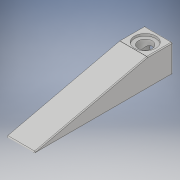
# Autodesk Inventor part: Wedge_base-left
Saved by Autodesk Inventor 2019.3 (Build 233278000, 278)
## iProperties
Created: 2019-02-07
Part Number: Wedge_base-left
Material: Generic
Document SubType Name: Modeling
Designer: Varga Daniel
Density: 1 g/cm^3
Appearance: Default
Author: Varga Daniel
Autodesk Inventor part; units mm, degrees
ref_plane "YZ Plane" through (0, 0, 0) normal (1, 0, 0) x (0, 1, 0)
ref_plane "XZ Plane" through (0, 0, 0) normal (0, 1, 0) x (-1, 0, 0)
ref_plane "XY Plane" through (0, 0, 0) normal (0, 0, 1) x (1, 0, 0)
derived "Connector_pin_base.ipt"
sketch "Pin_base_sketch" plane through (0, 0, 0) normal (0, 0, 1) x (1, 0, 0)
  line L0 (0, 0) -> (23.0918, 0) construction
  line L1 (0, 0) -> (0, 6.22) construction
  line L2 (0, 3.75) -> (0.563, 3.75)
  line L3 (0.863, 3.45) -> (0.863, 2.475)
  line L4 (0.863, 2.475) -> (9.988, 2.475)
  line L5 (9.988, 2.475) -> (9.988, 0)
  line L6 (0, 0) -> (0, 3.75)
  line L7 (0, 0) -> (9.988, 0)
  line L8 (9.288, 2.475) -> (9.288, 2.6)
  line L9 (9.988, 2.475) -> (9.988, 2.4774)
  arc A0 (9.988, 2.4774) -> (9.8454, 2.7031) centre (9.738, 2.4774) ccw
  arc A1 (9.8454, 2.7031) -> (9.288, 2.6) centre (9.6379, 2.267) ccw
  line L10 (9.8454, 2.7031) -> (9.8454, -0.0362) construction
  line L11 (8.9584, 2.75) -> (10.3858, 2.75) construction
  arc A2 (0.863, 3.45) -> (0.563, 3.75) centre (0.563, 3.45) ccw
  line L12 (0.863, 2.475) -> (0.863, 0)
  line L13 (-0.863, 2.475) -> (-0.863, 0)
  line L14 (-0.863, 3.45) -> (-0.863, 2.475)
  arc A3 (-0.563, 3.75) -> (-0.863, 3.45) centre (-0.563, 3.45) ccw
  line L15 (0, 3.75) -> (-0.563, 3.75)
  line L16 (0, 0) -> (-23.0918, 0) construction
  line L17 (0, 0) -> (-9.988, 0)
  line L18 (-0.863, 2.475) -> (-9.988, 2.475)
  line L19 (-9.288, 2.475) -> (-9.288, 2.6)
  arc A4 (-9.288, 2.6) -> (-9.8454, 2.7031) centre (-9.6379, 2.267) ccw
  arc A5 (-9.8454, 2.7031) -> (-9.988, 2.4774) centre (-9.738, 2.4774) ccw
  line L20 (-9.988, 2.475) -> (-9.988, 2.4774)
  line L21 (-8.9584, 2.75) -> (-10.3858, 2.75) construction
  line L22 (-9.8454, 2.7031) -> (-9.8454, -0.0362) construction
  line L23 (-9.988, 2.475) -> (-9.988, 0)
  line L24 (9.638, 3.1946) -> (9.638, -1.2485) construction
  dimension "d18" = 7.5
  dimension "d19" = 0.3
  dimension "d52" = 8.425
  dimension "d53" = 9.988
  measures "d18" diameter of L2 L0
  measures "d19" radius of A2
  measures "d52" distance between parallel lines of L19 L14
  measures "d53" distance between parallel lines of L23 L1
derived "Base_part.ipt"
sketch "Beam_sketch" plane through (0, 0, 0) normal (0, 1, 0) x (-1, 0, 0)
  line L0 (5, 0) -> (25, 0)
  line L1 (30, 5) -> (30, 25)
  line L2 (25, 30) -> (5, 30)
  line L3 (0, 25) -> (0, 5)
  line L4 (5, 29) -> (25, 29)
  line L5 (29, 25) -> (29, 5)
  line L6 (25, 1) -> (5, 1)
  line L7 (1, 5) -> (1, 25)
  circle A0 centre (5, 5) radius 2.5
  circle A1 centre (5, 5) radius 3.5
  arc A2 (25, 0) -> (30, 5) centre (25, 5) ccw
  arc A3 (30, 25) -> (25, 30) centre (25, 25) ccw
  arc A4 (5, 30) -> (0, 25) centre (5, 25) ccw
  arc A5 (0, 5) -> (5, 0) centre (5, 5) ccw
  arc A6 (1, 5) -> (5, 1) centre (5, 5) ccw
  arc A7 (5, 29) -> (1, 25) centre (5, 25) ccw
  arc A8 (29, 25) -> (25, 29) centre (25, 25) ccw
  arc A9 (25, 1) -> (29, 5) centre (25, 5) ccw
  line L8 (49.1041, 15) -> (-27.081, 15) construction
  line L9 (31.1478, 10) -> (-2.4877, 10) construction
  line L10 (-2.8604, 5) -> (35.495, 5) construction
  line L11 (5, -2.5736) -> (5, 36.7522) construction
  line L12 (15, -1.4978) -> (15, 34.8784) construction
  line L13 (1.5359, 5.5) -> (1, 5.5)
  line L14 (1.5359, 4.5) -> (1.0314, 4.5)
  line L15 (28.9686, 4.5) -> (8.4641, 4.5)
  line L16 (29, 5.5) -> (8.4641, 5.5)
  line L17 (4.5, 1.5359) -> (4.5, 1.0314)
  line L18 (5.5, 1.5359) -> (5.5, 1)
  line L19 (29, 10.5) -> (1, 10.5)
  line L20 (29, 9.5) -> (1, 9.5)
  line L21 (4.5, 28.9686) -> (4.5, 10.5)
  line L22 (4.5, 9.5) -> (4.5, 8.4641)
  line L23 (5.5, 29) -> (5.5, 10.5)
  line L24 (5.5, 9.5) -> (5.5, 8.4641)
  point P0 (0, 0)
  point P1 (30, 30)
  point P2 (0, 30)
  dimension "d1" = 7
  dimension "d2" = 5
  measures "d2" diameter of A0
sketch "Sketch2" plane through (0, 0, 0) normal (1, 0, 0) x (0, 1, 0)
  line L0 (0, 0) -> (10, 0)
  line L1 (10, 0) -> (10, 9.2)
  line L2 (10, 9.2) -> (0.5922, 49.7678)
  line L3 (0, 49.7) -> (0, 0)
  line L4 (0, 47.895) -> (8.9735, 9.2)
  line L5 (8.9735, 9.2) -> (0, 9.2)
  arc A0 (0.5922, 49.7678) -> (0, 49.7) centre (0.3, 49.7) ccw
  point P0 (0, 52.3216)
  dimension "d3" = 10
  dimension "d5" = 1
  dimension "d6" = 9.2
  dimension "d38" = 0.3
  dimension "d39" = 50
  constraints: 12 end point, 5 point on line, 2 parallel, 2 perpendicular, 2 point on circle, 2 tangent, 1 centre point, 1 horizontal
  measures "d3" distance between parallel lines of L1 L3
  measures "d5" distance between parallel lines of L2 L4
  measures "d6" distance between parallel lines of L5 L0
  measures "d38" radius of A0
extrude "Extrusion1" add sketch "Sketch2" against normal blind 10 contours L3 L5 L4 A0 L2 L1 L0
extrude "Left_wall" add sketch "Sketch2" against normal blind 1 contours L3 L4 L5
sketch "Sketch3" plane through (-10, 0, 0) normal (-1, 0, 0) x (0, 0, 1)
  line L0 (9.2, 8.9735) -> (9.2, 0) projected
  line L1 (47.895, 0) -> (9.2, 8.9735) projected
  line L2 (49.7, 0) -> (0, 0) projected
  point P0 (50, 0)
extrude "Right_wall" [suppressed]
sketch "Sketch4" plane through (-10, 0, 0) normal (0, -1, 0) x (1, 0, 0)
  line L0 (9, 47.895) -> (0, 47.895) construction
  line L1 (9, 9.2) -> (0, 9.2) construction
  line L2 (10, 0) -> (0, 0) construction
  line L3 (10, 49.7) -> (10, 0) construction
  circle A0 centre (5, 5) radius 3.85
  circle A1 centre (5, 5) radius 2.5
  line L4 (10, 49.7) -> (0, 49.7) projected
  line L5 (0, 47.895) -> (0, 49.7) projected
  line L6 (9, 9.2) -> (9, 47.895) projected
  line L7 (0, 0) -> (0, 9.2) projected
  dimension "d14" = 5
  dimension "d15" = 5
  dimension "d16" = 7.7
  dimension "d49" = 5
  constraints: 2 centre point, 1 coincident
  measures "d14" distance from line of A0.centre L2
  measures "d15" diameter of A1
  measures "d16" diameter of A0
  measures "d49" distance from line of A0.centre L3
extrude "Extrusion4" cut sketch "Sketch4" against normal through all contours A1
extrude "Extrusion6" cut sketch "Sketch4" against normal blind 0.8
sketch "Sketch6" plane through (0, 10, 9.2) normal (0, 1, 0) x (1, 0, 0)
  circle A0 centre (-5, 4.2) radius 3.85 projected
  circle A1 centre (-5, 4.2) radius 2.5 projected
  point P0 (0, 9.2)
extrude "Extrusion7" cut sketch "Sketch6" against normal blind 0.8
sketch "Sketch10" plane through (0, 0, 0) normal (0, 0, -1) x (-1, 0, 0)
  line L0 (0, 0) -> (0, 10) construction
  line L1 (0, 0) -> (10, 0) construction
  line L2 (10, 10) -> (10, 0) construction
  line L3 (0, 10) -> (10, 10) construction
  circle A0 centre (5, 5) radius 2.5
  circle A1 centre (5, 5) radius 3.85
  dimension "d43" = 5
  dimension "d44" = 7.7
  dimension "d45" = 5
  dimension "d46" = 5
  constraints: 2 centre point, 1 coincident
  measures "d43" diameter of A0
  measures "d44" diameter of A1
  measures "d45" distance from line of A0.centre L2
  measures "d46" distance from line of A0.centre L1
extrude "Extrusion11" cut sketch "Sketch10" against normal up to surface (9.2 mm away) contours A0
extrude "Extrusion12" cut sketch "Sketch10" against normal blind 0.8
fillet "Fillet1" radius 0.3 3 edges at (-5, 10, 0) (-5, 0, 0) (-5, 10, 9.2)
fillet "Left_fillet" radius 0.3 8 edges at (0, 9.9981, 9.1998) (0, 5.2922, 29.5006) (0, 0.2659, 49.9981) (0, 0, 25) (0, 0.0879, 0.0879) (0, 5, 0) (0, 9.9121, 0.0879) (0, 10, 4.7328)
fillet "Right_fillet" [suppressed]
equation "\"d5\" = Wall_thickness"
equation "\"d6\" = 0.5 * Overall_height + 0.5 * Hole_height"
equation "\"d38\" = Wedge_end_fillet_radius"
equation "\"d39\" = Wedge_length"
equation "\"d9\" = Wall_thickness"
equation "\"d11\" = Wall_thickness"
equation "\"d15\" = d2"
equation "\"d16\" = d18 + Wedge_Pin_collar_diameter_tolerance"
equation "\"d20\" = Wall_thickness"
equation "\"d24\" = -0.5 * Hole_height + 0.5 * Overall_height"
equation "\"d26\" = -0.5 * Hole_height + 0.5 * Overall_height"
equation "\"d43\" = d15"
equation "\"d44\" = d16"
equation "\"d50\" = -0.5 * Hole_height + 0.5 * Overall_height"
equation "\"d40\" = Wedge_fillet_radius"
equation "\"d41\" = Wedge_fillet_radius"
equation "\"d42\" = Wedge_fillet_radius"
equation "\"Wedge_Pin_collar_diameter_tolerance\" = 0.2"
equation "\"Wedge_end_fillet_radius\" = 0.3"
equation "\"Wedge_wall_thickness\" = Wall_thickness"
equation "\"Wedge_fillet_radius\" = 0.3"
equation "\"Wall_thickness\" = 1"
equation "\"Overall_height\" = 10"
equation "\"Hole_height\" = 8.4"
equation "\"Wedge_length\" = 50"
body "Solid1"
